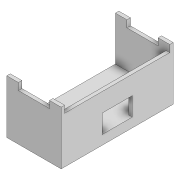
# Autodesk Inventor part: US_Casis
Saved by Autodesk Inventor 2021 (Build 250183000, 183)
## iProperties
Created: 2021-03-20
Part Number: US_Casis
Material: Generic
Document SubType Name: Modeling
Designer: Kyler Martinez
Density: 1 g/cm^3
Appearance: Default
Author: Kyler Martinez
Autodesk Inventor part; units mm, degrees
ref_plane "YZ Plane" through (0, 0, 0) normal (1, 0, 0) x (0, 1, 0)
ref_plane "XZ Plane" through (0, 0, 0) normal (0, 1, 0) x (-1, 0, 0)
ref_plane "XY Plane" through (0, 0, 0) normal (0, 0, 1) x (1, 0, 0)
sketch "Sketch1" plane through (0, 0, 0) normal (0, 1, 0) x (-1, 0, 0)
  line L0 (-6.6677, 20.126) -> (13.7323, 20.126)
  line L1 (13.7323, 20.126) -> (13.7323, -25.074)
  line L2 (13.7323, -25.074) -> (-6.6677, -25.074)
  line L3 (-6.6677, -25.074) -> (-6.6677, 20.126)
  line L4 (15.2323, -26.574) -> (15.2323, 21.626)
  line L5 (15.2323, 21.626) -> (-8.1677, 21.626)
  line L6 (-8.1677, 21.626) -> (-8.1677, -26.574)
  line L7 (-8.1677, -26.574) -> (15.2323, -26.574)
  point P0 (0, 0)
  dimension "d0" = 45.2
  dimension "d1" = 20.4
  dimension "d2" = 1.5
  constraints: 16 end point, 4 parallel, 2 perpendicular, 1 horizontal, 3 other
  measures "d0" distance of L0.end L1.end
  measures "d1" distance of L1.end L2.end
  measures "d2" distance between parallel lines of L1 L4
extrude "Extrusion1" add sketch "Sketch1" along normal blind 20
sketch "Sketch2" plane through (8.1677, 0, 21.626) normal (1, 0, 0) x (0, 0, -1)
  line L0 (19.1022, 10.5) -> (29.1022, 10.5)
  line L1 (29.1022, 10.5) -> (29.1022, 5.5)
  line L2 (29.1022, 5.5) -> (19.1022, 5.5)
  line L3 (19.1022, 5.5) -> (19.1022, 10.5)
  line L4 (30.6022, 12) -> (17.6022, 12)
  line L5 (17.6022, 12) -> (17.6022, 4)
  line L6 (17.6022, 4) -> (30.6022, 4)
  line L7 (30.6022, 4) -> (30.6022, 12)
  line L8 (0, 0) -> (0, 20) projected
  line L9 (48.2, 0) -> (48.2, 20) projected
  line L10 (0, 20) -> (48.2, 20) projected
  point P0 (21.626, 0)
  dimension "d5" = 10
  dimension "d6" = 5
  dimension "d7" = 1.5
  dimension "d8" = 17.6022
  dimension "d9" = 17.5978
  dimension "d10" = 8
  constraints: 16 end point, 4 parallel, 2 perpendicular, 1 horizontal, 3 other
  measures "d5" distance of L1.end L2.end
  measures "d6" distance of L0.end L1.end
  measures "d7" distance between parallel lines of L0 L4
  measures "d8" distance between parallel lines of L8 L5
  measures "d9" distance between parallel lines of L9 L7
  measures "d10" distance between parallel lines of L4 L10
extrude "Extrusion2" cut sketch "Sketch2" against normal blind 6 contours L0 L1 L2 L3 | L7 L6 L5 L4
extrude "Extrusion3" add sketch "Sketch1" along normal blind 4 contours L0 L1 L2 L3
sketch "Sketch3" plane through (0, 20, 0) normal (0, 1, 0) x (1, 0, 0)
  line L0 (-13.7323, -20.126) -> (-13.7323, 25.074) projected
  line L1 (-15.2323, 26.574) -> (-15.2323, -21.626) projected
  line L2 (-13.7323, -20.126) -> (-15.2323, -20.126)
  line L3 (-15.2323, -20.126) -> (-15.2323, 25.074)
  line L4 (-15.2323, 25.074) -> (-13.7323, 25.074)
  line L5 (-13.7323, 25.074) -> (-13.7323, -20.126)
  point P0 (0, 0)
  dimension "d17" = 0
  constraints: 8 end point, 2 parallel, 1 horizontal, 1 perpendicular, 1 point on line
  measures "d17" distance from line of L0.end L4
extrude "Extrusion4" cut sketch "Sketch3" against normal blind 16
sketch "Sketch4" plane through (0, 20, 0) normal (0, 1, 0) x (1, 0, 0)
  line L0 (-15.2323, -20.126) -> (-15.2323, -21.626) projected
  line L1 (-15.2323, -21.626) -> (8.1677, -21.626) projected
  line L2 (-15.2323, -20.126) -> (-10.2323, -20.126)
  line L3 (-10.2323, -20.126) -> (-10.2323, -21.626)
  line L4 (-10.2323, -21.626) -> (-15.2323, -21.626)
  line L5 (-15.2323, -21.626) -> (-15.2323, -20.126)
  line L6 (6.6677, -20.126) -> (-15.2323, -20.126) projected
  line L7 (8.1677, -21.626) -> (3.1677, -21.626)
  line L8 (3.1677, -21.626) -> (3.1677, -20.126)
  line L9 (3.1677, -20.126) -> (8.1677, -20.126)
  line L10 (8.1677, -20.126) -> (8.1677, -21.626)
  line L11 (8.1677, 26.574) -> (-15.2323, 26.574) projected
  line L12 (-15.2323, 25.074) -> (6.6677, 25.074) projected
  line L13 (-15.2323, 26.574) -> (-10.2323, 26.574)
  line L14 (-10.2323, 26.574) -> (-10.2323, 25.074)
  line L15 (-10.2323, 25.074) -> (-15.2323, 25.074)
  line L16 (-15.2323, 25.074) -> (-15.2323, 26.574)
  line L17 (8.1677, -21.626) -> (8.1677, 26.574) projected
  line L18 (8.1677, 26.574) -> (3.1677, 26.574)
  line L19 (3.1677, 26.574) -> (3.1677, 25.074)
  line L20 (3.1677, 25.074) -> (8.1677, 25.074)
  line L21 (8.1677, 25.074) -> (8.1677, 26.574)
  point P0 (0, 0)
  dimension "d18" = 5
  dimension "d19" = 5
  dimension "d20" = 5
  dimension "d21" = 5
  constraints: 32 end point, 8 parallel, 4 horizontal, 4 perpendicular, 4 point on line
  measures "d18" distance of L0.start L2.end
  measures "d19" distance of L8.end L9.end
  measures "d20" distance of L14.end L15.end
  measures "d21" distance of L20.end L19.end
extrude "Extrusion5" add sketch "Sketch4" along normal blind 3 contours L2 L3 L1 L0 | L20 L12 L19 L11 L17 | L6 L9 L10 L1 L8 | L14 L12 L16 L11
body "Solid1"
